Autodesk Fusion 360 part; units mm, degrees
(part 15 of 21)
  spline S63 degree 3 poles (-9.8498, -24.8525) (-9.8587, -24.8489) (-9.8682, -24.8467) (-9.8874, -24.845) (-9.8971, -24.8455) (-9.9193, -24.85) (-9.9314, -24.8551) (-9.9531, -24.8696) (-9.9624, -24.8789) (-9.9696, -24.8897) knots -0.013599 -0.013599 -0.013599 -0.013599 -0.010706 -0.010706 -0.007813 -0.007813 -0.003906 -0.003906 0 0 0 0
  arc A33 (-9.8498, -24.8525) -> (-9.3097, -25.0598) centre (0, 0) ccw
  spline S64 degree 3 poles (-9.2456, -25.1676) (-9.2442, -25.1581) (-9.2442, -25.1484) (-9.2471, -25.1293) (-9.2499, -25.12) (-9.2594, -25.0995) (-9.2672, -25.0888) (-9.2863, -25.0712) (-9.2975, -25.0643) (-9.3097, -25.0598) knots -0.013599 -0.013599 -0.013599 -0.013599 -0.010706 -0.010706 -0.007813 -0.007813 -0.003906 -0.003906 0 0 0 0
  spline S65 degree 3 poles (-9.2557, -27.3039) (-9.2937, -26.9335) (-9.315, -26.5537) (-9.3122, -25.8487) (-9.2928, -25.4995) (-9.2456, -25.1676) knots -0.220678 -0.220678 -0.220678 -0.220678 -0.107909 -0.107909 -0.008028 -0.008028 -0.008028 -0.008028
  arc A34 (-9.2557, -27.3039) -> (-8.5608, -27.5296) centre (0, 0) ccw
  spline S66 degree 3 poles (-7.3133, -25.7954) (-7.4702, -26.0917) (-7.6598, -26.3856) (-8.0719, -26.9576) (-8.3124, -27.2523) (-8.5608, -27.5296) knots -0.210627 -0.210627 -0.210627 -0.210627 -0.111696 -0.111696 0 0 0 0
  spline S67 degree 3 poles (-7.198, -25.7459) (-7.2073, -25.7433) (-7.2169, -25.7421) (-7.2362, -25.7424) (-7.2458, -25.7439) (-7.2674, -25.7508) (-7.2789, -25.757) (-7.2989, -25.7737) (-7.3072, -25.7839) (-7.3133, -25.7954) knots -0.013599 -0.013599 -0.013599 -0.013599 -0.010706 -0.010706 -0.007813 -0.007813 -0.003906 -0.003906 0 0 0 0
  arc A35 (-7.198, -25.7459) -> (-6.6393, -25.8956) centre (0, 0) ccw
  spline S68 degree 3 poles (-6.5642, -25.9962) (-6.5638, -25.9865) (-6.5649, -25.9769) (-6.5697, -25.9582) (-6.5734, -25.9493) (-6.5851, -25.9298) (-6.5939, -25.9201) (-6.6148, -25.9045) (-6.6267, -25.8989) (-6.6393, -25.8956) knots -0.013599 -0.013599 -0.013599 -0.013599 -0.010706 -0.010706 -0.007813 -0.007813 -0.003906 -0.003906 0 0 0 0
  spline S69 degree 3 poles (-6.351, -28.1218) (-6.4275, -27.7574) (-6.4884, -27.3819) (-6.5592, -26.6805) (-6.5765, -26.3312) (-6.5642, -25.9962) knots -0.220678 -0.220678 -0.220678 -0.220678 -0.107909 -0.107909 -0.008028 -0.008028 -0.008028 -0.008028
  arc A36 (-6.351, -28.1218) -> (-5.6363, -28.2737) centre (0, 0) ccw
  spline S70 degree 3 poles (-4.5769, -26.4186) (-4.702, -26.7296) (-4.8598, -27.0417) (-5.2098, -27.6537) (-5.4182, -27.9719) (-5.6363, -28.2737) knots -0.210627 -0.210627 -0.210627 -0.210627 -0.111696 -0.111696 0 0 0 0
  spline S71 degree 3 poles (-4.4674, -26.3573) (-4.4769, -26.3557) (-4.4866, -26.3554) (-4.5058, -26.3578) (-4.5151, -26.3603) (-4.5359, -26.3693) (-4.5467, -26.3768) (-4.5649, -26.3955) (-4.572, -26.4065) (-4.5769, -26.4186) knots -0.013599 -0.013599 -0.013599 -0.013599 -0.010706 -0.010706 -0.007813 -0.007813 -0.003906 -0.003906 0 0 0 0
  arc A37 (-4.4674, -26.3573) -> (-3.8961, -26.4478) centre (0, 0) ccw
  spline S72 degree 3 poles (-3.8109, -26.5399) (-3.8115, -26.5303) (-3.8136, -26.5208) (-3.8203, -26.5027) (-3.825, -26.4942) (-3.8386, -26.4761) (-3.8484, -26.4674) (-3.8708, -26.4541) (-3.8832, -26.4497) (-3.8961, -26.4478) knots -0.013599 -0.013599 -0.013599 -0.013599 -0.010706 -0.010706 -0.007813 -0.007813 -0.003906 -0.003906 0 0 0 0
  spline S73 degree 3 poles (-3.3766, -28.6316) (-3.4908, -28.2772) (-3.5906, -27.9101) (-3.7344, -27.2199) (-3.7881, -26.8744) (-3.8109, -26.5399) knots -0.220678 -0.220678 -0.220678 -0.220678 -0.107909 -0.107909 -0.008028 -0.008028 -0.008028 -0.008028
  arc A38 (-3.3766, -28.6316) -> (-2.65, -28.708) centre (0, 0) ccw
  spline S74 degree 3 poles (-1.7903, -26.7523) (-1.8822, -27.0747) (-2.0065, -27.4015) (-2.2907, -28.0467) (-2.4646, -28.385) (-2.65, -28.708) knots -0.210627 -0.210627 -0.210627 -0.210627 -0.111696 -0.111696 0 0 0 0
  spline S75 degree 3 poles (-1.6879, -26.6799) (-1.6975, -26.6793) (-1.7071, -26.68) (-1.7259, -26.6844) (-1.735, -26.6879) (-1.7547, -26.699) (-1.7647, -26.7076) (-1.7808, -26.728) (-1.7868, -26.7397) (-1.7903, -26.7523) knots -0.013599 -0.013599 -0.013599 -0.013599 -0.010706 -0.010706 -0.007813 -0.007813 -0.003906 -0.003906 0 0 0 0
  arc A39 (-1.6879, -26.6799) -> (-1.1102, -26.7101) centre (0, 0) ccw
  spline S76 degree 3 poles (-1.0158, -26.7929) (-1.0175, -26.7834) (-1.0205, -26.7741) (-1.0291, -26.7569) (-1.0346, -26.7489) (-1.0501, -26.7323) (-1.0607, -26.7246) (-1.0844, -26.7138) (-1.0972, -26.7107) (-1.1102, -26.7101) knots -0.013599 -0.013599 -0.013599 -0.013599 -0.010706 -0.010706 -0.007813 -0.007813 -0.003906 -0.003906 0 0 0 0
  spline S77 degree 3 poles (-0.3653, -28.8277) (-0.5159, -28.4872) (-0.6536, -28.1325) (-0.8687, -27.4612) (-0.9582, -27.1231) (-1.0158, -26.7929) knots -0.220678 -0.220678 -0.220678 -0.220678 -0.107909 -0.107909 -0.008028 -0.008028 -0.008028 -0.008028
  arc A40 (-0.3653, -28.8277) -> (0.3653, -28.8277) centre (0, 0) ccw
  spline S78 degree 3 poles (1.0158, -26.7929) (0.9582, -27.1231) (0.8687, -27.4612) (0.6536, -28.1325) (0.5159, -28.4872) (0.3653, -28.8277) knots -0.210627 -0.210627 -0.210627 -0.210627 -0.111696 -0.111696 0 0 0 0
  spline S79 degree 3 poles (1.1102, -26.7101) (1.1006, -26.7105) (1.091, -26.7123) (1.0728, -26.7186) (1.0642, -26.723) (1.0457, -26.7362) (1.0367, -26.7457) (1.0228, -26.7678) (1.0181, -26.78) (1.0158, -26.7929) knots -0.013599 -0.013599 -0.013599 -0.013599 -0.010706 -0.010706 -0.007813 -0.007813 -0.003906 -0.003906 0 0 0 0
  arc A41 (1.1102, -26.7101) -> (1.6879, -26.6799) centre (0, 0) ccw
  spline S80 degree 3 poles (1.7903, -26.7523) (1.7877, -26.743) (1.7837, -26.7341) (1.7734, -26.7179) (1.7671, -26.7105) (1.75, -26.6957) (1.7386, -26.6891) (1.7139, -26.6808) (1.7008, -26.679) (1.6879, -26.6799) knots -0.013599 -0.013599 -0.013599 -0.013599 -0.010706 -0.010706 -0.007813 -0.007813 -0.003906 -0.003906 0 0 0 0
  spline S81 degree 3 poles (2.65, -28.708) (2.4646, -28.385) (2.2907, -28.0467) (2.0065, -27.4015) (1.8822, -27.0747) (1.7903, -26.7523) knots -0.220678 -0.220678 -0.220678 -0.220678 -0.107909 -0.107909 -0.008028 -0.008028 -0.008028 -0.008028
  arc A42 (2.65, -28.708) -> (3.3766, -28.6316) centre (0, 0) ccw
  spline S82 degree 3 poles (3.8109, -26.5399) (3.7881, -26.8744) (3.7344, -27.2199) (3.5906, -27.9101) (3.4908, -28.2772) (3.3766, -28.6316) knots -0.210627 -0.210627 -0.210627 -0.210627 -0.111696 -0.111696 0 0 0 0
  spline S83 degree 3 poles (3.8961, -26.4478) (3.8865, -26.4492) (3.8773, -26.452) (3.8598, -26.4601) (3.8517, -26.4654) (3.8347, -26.4804) (3.8267, -26.4908) (3.8152, -26.5142) (3.8118, -26.5269) (3.8109, -26.5399) knots -0.013599 -0.013599 -0.013599 -0.013599 -0.010706 -0.010706 -0.007813 -0.007813 -0.003906 -0.003906 0 0 0 0
  arc A43 (3.8961, -26.4478) -> (4.4674, -26.3573) centre (0, 0) ccw
  spline S84 degree 3 poles (4.5769, -26.4186) (4.5733, -26.4096) (4.5684, -26.4012) (4.5564, -26.3861) (4.5494, -26.3795) (4.5308, -26.3665) (4.5188, -26.3612) (4.4934, -26.3555) (4.4803, -26.3551) (4.4674, -26.3573) knots -0.013599 -0.013599 -0.013599 -0.013599 -0.010706 -0.010706 -0.007813 -0.007813 -0.003906 -0.003906 0 0 0 0
  spline S85 degree 3 poles (5.6363, -28.2737) (5.4182, -27.9719) (5.2098, -27.6537) (4.8598, -27.0417) (4.702, -26.7296) (4.5769, -26.4186) knots -0.220678 -0.220678 -0.220678 -0.220678 -0.107909 -0.107909 -0.008028 -0.008028 -0.008028 -0.008028
  arc A44 (5.6363, -28.2737) -> (6.351, -28.1218) centre (0, 0) ccw
  spline S86 degree 3 poles (6.5642, -25.9962) (6.5765, -26.3312) (6.5592, -26.6805) (6.4884, -27.3819) (6.4275, -27.7574) (6.351, -28.1218) knots -0.210627 -0.210627 -0.210627 -0.210627 -0.111696 -0.111696 0 0 0 0
  spline S87 degree 3 poles (6.6393, -25.8956) (6.6299, -25.898) (6.621, -25.9018) (6.6045, -25.9117) (6.5969, -25.9178) (6.5816, -25.9345) (6.5748, -25.9457) (6.5658, -25.9702) (6.5637, -25.9831) (6.5642, -25.9962) knots -0.013599 -0.013599 -0.013599 -0.013599 -0.010706 -0.010706 -0.007813 -0.007813 -0.003906 -0.003906 0 0 0 0
  arc A45 (6.6393, -25.8956) -> (7.198, -25.7459) centre (0, 0) ccw
  spline S88 degree 3 poles (7.3133, -25.7954) (7.3088, -25.7869) (7.3031, -25.7791) (7.2896, -25.7653) (7.2819, -25.7594) (7.2621, -25.7485) (7.2495, -25.7444) (7.2237, -25.7414) (7.2106, -25.7424) (7.198, -25.7459) knots -0.013599 -0.013599 -0.013599 -0.013599 -0.010706 -0.010706 -0.007813 -0.007813 -0.003906 -0.003906 0 0 0 0
  spline S89 degree 3 poles (8.5608, -27.5296) (8.3124, -27.2523) (8.0719, -26.9576) (7.6598, -26.3856) (7.4702, -26.0917) (7.3133, -25.7954) knots -0.220678 -0.220678 -0.220678 -0.220678 -0.107909 -0.107909 -0.008028 -0.008028 -0.008028 -0.008028
  arc A46 (8.5608, -27.5296) -> (9.2557, -27.3039) centre (0, 0) ccw
  spline S90 degree 3 poles (9.2456, -25.1676) (9.2928, -25.4995) (9.3122, -25.8487) (9.315, -26.5537) (9.2937, -26.9335) (9.2557, -27.3039) knots -0.210627 -0.210627 -0.210627 -0.210627 -0.111696 -0.111696 0 0 0 0
  spline S91 degree 3 poles (9.3097, -25.0598) (9.3007, -25.0631) (9.2922, -25.0678) (9.2768, -25.0794) (9.27, -25.0863) (9.2565, -25.1045) (9.2508, -25.1163) (9.2444, -25.1416) (9.2437, -25.1547) (9.2456, -25.1676) knots -0.013599 -0.013599 -0.013599 -0.013599 -0.010706 -0.010706 -0.007813 -0.007813 -0.003906 -0.003906 0 0 0 0
  arc A47 (9.3097, -25.0598) -> (9.8498, -24.8525) centre (0, 0) ccw
  spline S92 degree 3 poles (9.9696, -24.8897) (9.9642, -24.8817) (9.9577, -24.8745) (9.9429, -24.8622) (9.9346, -24.8572) (9.9137, -24.8483) (9.9008, -24.8456) (9.8748, -24.8453) (9.8619, -24.8477) (9.8498, -24.8525) knots -0.013599 -0.013599 -0.013599 -0.013599 -0.010706 -0.010706 -0.007813 -0.007813 -0.003906 -0.003906 0 0 0 0
  spline S93 degree 3 poles (11.3915, -26.484) (11.1155, -26.2342) (10.8455, -25.9662) (10.3759, -25.4404) (10.1566, -25.1679) (9.9696, -24.8897) knots -0.220678 -0.220678 -0.220678 -0.220678 -0.107909 -0.107909 -0.008028 -0.008028 -0.008028 -0.008028
  arc A48 (11.3915, -26.484) -> (12.059, -26.1868) centre (0, 0) ccw
  spline S94 degree 3 poles (11.8257, -24.0633) (11.9073, -24.3884) (11.9631, -24.7337) (12.0396, -25.4345) (12.0581, -25.8145) (12.059, -26.1868) knots -0.210627 -0.210627 -0.210627 -0.210627 -0.111696 -0.111696 0 0 0 0
  spline S95 degree 3 poles (11.8782, -23.9494) (11.8696, -23.9537) (11.8616, -23.9592) (11.8475, -23.9723) (11.8414, -23.9799) (11.8299, -23.9994) (11.8255, -24.0118) (11.8218, -24.0376) (11.8225, -24.0507) (11.8257, -24.0633) knots -0.013599 -0.013599 -0.013599 -0.013599 -0.010706 -0.010706 -0.007813 -0.007813 -0.003906 -0.003906 0 0 0 0
  arc A49 (11.8782, -23.9494) -> (12.3936, -23.6868) centre (0, 0) ccw
  spline S96 degree 3 poles (12.5167, -23.7112) (12.5105, -23.7038) (12.5033, -23.6974) (12.4872, -23.6867) (12.4784, -23.6826) (12.4568, -23.6759) (12.4437, -23.6746) (12.4178, -23.677) (12.4051, -23.6807) (12.3936, -23.6868) knots -0.013599 -0.013599 -0.013599 -0.013599 -0.010706 -0.010706 -0.007813 -0.007813 -0.003906 -0.003906 0 0 0 0
  spline S97 degree 3 poles (14.0975, -25.1482) (13.7968, -24.9286) (13.5003, -24.6903) (12.9783, -24.2164) (12.7317, -23.9684) (12.5167, -23.7112) knots -0.220678 -0.220678 -0.220678 -0.220678 -0.107909 -0.107909 -0.008028 -0.008028 -0.008028 -0.008028
  arc A50 (14.0975, -25.1482) -> (14.7302, -24.7828) centre (0, 0) ccw
  spline S98 degree 3 poles (14.2762, -22.6954) (14.3914, -23.0102) (14.4829, -23.3477) (14.6323, -24.0367) (14.6904, -24.4127) (14.7302, -24.7828) knots -0.210627 -0.210627 -0.210627 -0.210627 -0.111696 -0.111696 0 0 0 0
  spline S99 degree 3 poles (14.3165, -22.5766) (14.3084, -22.5817) (14.301, -22.588) (14.2884, -22.6026) (14.2831, -22.6107) (14.2737, -22.6313) (14.2707, -22.6441) (14.2697, -22.6702) (14.2717, -22.6831) (14.2762, -22.6954) knots -0.013599 -0.013599 -0.013599 -0.013599 -0.010706 -0.010706 -0.007813 -0.007813 -0.003906 -0.003906 0 0 0 0
  arc A51 (14.3165, -22.5766) -> (14.8017, -22.2615) centre (0, 0) ccw
  spline S100 degree 3 poles (14.9266, -22.273) (14.9197, -22.2663) (14.9118, -22.2606) (14.8947, -22.2517) (14.8856, -22.2485) (14.8633, -22.2441) (14.8502, -22.2442) (14.8246, -22.2493) (14.8125, -22.2543) (14.8017, -22.2615) knots -0.013599 -0.013599 -0.013599 -0.013599 -0.010706 -0.010706 -0.007813 -0.007813 -0.003906 -0.003906 0 0 0 0
  spline S101 degree 3 poles (16.6489, -23.5368) (16.327, -23.3499) (16.0071, -23.1439) (15.4385, -22.7272) (15.1674, -22.5063) (14.9266, -22.273) knots -0.220678 -0.220678 -0.220678 -0.220678 -0.107909 -0.107909 -0.008028 -0.008028 -0.008028 -0.008028
  arc A52 (16.6489, -23.5368) -> (17.24, -23.1074) centre (0, 0) ccw
  spline S102 degree 3 poles (16.5703, -21.0788) (16.7177, -21.3798) (16.8441, -21.7059) (17.0646, -22.3755) (17.1617, -22.7434) (17.24, -23.1074) knots -0.210627 -0.210627 -0.210627 -0.210627 -0.111696 -0.111696 0 0 0 0
  spline S103 degree 3 poles (16.598, -20.9564) (16.5904, -20.9624) (16.5838, -20.9694) (16.5727, -20.9852) (16.5683, -20.9939) (16.5611, -21.0154) (16.5594, -21.0284) (16.5612, -21.0544) (16.5645, -21.0671) (16.5703, -21.0788) knots -0.013599 -0.013599 -0.013599 -0.013599 -0.010706 -0.010706 -0.007813 -0.007813 -0.003906 -0.003906 0 0 0 0
  arc A53 (16.598, -20.9564) -> (17.0475, -20.5924) centre (0, 0) ccw
  spline S104 degree 3 poles (17.173, -20.5907) (17.1654, -20.5848) (17.157, -20.5799) (17.1391, -20.5728) (17.1296, -20.5706) (17.1071, -20.5686) (17.094, -20.5701) (17.0691, -20.5778) (17.0576, -20.5841) (17.0475, -20.5924) knots -0.013599 -0.013599 -0.013599 -0.013599 -0.010706 -0.010706 -0.007813 -0.007813 -0.003906 -0.003906 0 0 0 0
  spline S105 degree 3 poles (19.018, -21.6676) (18.6782, -21.5153) (18.3387, -21.3439) (17.7295, -20.9889) (17.4368, -20.7975) (17.173, -20.5907) knots -0.220678 -0.220678 -0.220678 -0.220678 -0.107909 -0.107909 -0.008028 -0.008028 -0.008028 -0.008028
  arc A54 (19.018, -21.6676) -> (19.561, -21.1787) centre (0, 0) ccw
  spline S106 degree 3 poles (18.6828, -19.2312) (18.861, -19.5152) (19.0207, -19.8263) (19.31, -20.4692) (19.445, -20.8249) (19.561, -21.1787) knots -0.210627 -0.210627 -0.210627 -0.210627 -0.111696 -0.111696 0 0 0 0
  spline S107 degree 3 poles (18.6976, -19.1066) (18.6907, -19.1134) (18.6848, -19.1211) (18.6755, -19.1379) (18.672, -19.147) (18.6671, -19.1691) (18.6668, -19.1823) (18.6712, -19.2079) (18.6759, -19.2202) (18.6828, -19.2312) knots -0.013599 -0.013599 -0.013599 -0.013599 -0.010706 -0.010706 -0.007813 -0.007813 -0.003906 -0.003906 0 0 0 0
  arc A55 (18.6976, -19.1066) -> (19.1066, -18.6976) centre (0, 0) ccw
  spline S108 degree 3 poles (19.2312, -18.6828) (19.2231, -18.6777) (19.2142, -18.6738) (19.1956, -18.6686) (19.186, -18.6674) (19.1633, -18.6678) (19.1505, -18.6706) (19.1266, -18.6809) (19.1157, -18.6883) (19.1066, -18.6976) knots -0.013599 -0.013599 -0.013599 -0.013599 -0.010706 -0.010706 -0.007813 -0.007813 -0.003906 -0.003906 0 0 0 0
  spline S109 degree 3 poles (21.1787, -19.561) (20.8249, -19.445) (20.4692, -19.31) (19.8263, -19.0207) (19.5152, -18.861) (19.2312, -18.6828) knots -0.220678 -0.220678 -0.220678 -0.220678 -0.107909 -0.107909 -0.008028 -0.008028 -0.008028 -0.008028
  arc A56 (21.1787, -19.561) -> (21.6676, -19.018) centre (0, 0) ccw
  spline S110 degree 3 poles (20.5907, -17.173) (20.7975, -17.4368) (20.9889, -17.7295) (21.3439, -18.3387) (21.5153, -18.6782) (21.6676, -19.018) knots -0.210627 -0.210627 -0.210627 -0.210627 -0.111696 -0.111696 0 0 0 0
  spline S111 degree 3 poles (20.5924, -17.0475) (20.5862, -17.055) (20.5812, -17.0632) (20.5736, -17.081) (20.5711, -17.0904) (20.5686, -17.1129) (20.5696, -17.126) (20.5767, -17.151) (20.5827, -17.1628) (20.5907, -17.173) knots -0.013599 -0.013599 -0.013599 -0.013599 -0.010706 -0.010706 -0.007813 -0.007813 -0.003906 -0.003906 0 0 0 0
  arc A57 (20.5924, -17.0475) -> (20.9564, -16.598) centre (0, 0) ccw
  spline S112 degree 3 poles (21.0788, -16.5703) (21.0701, -16.566) (21.0609, -16.5631) (21.0419, -16.5599) (21.0322, -16.5597) (21.0097, -16.5624) (20.9972, -16.5665) (20.9745, -16.5793) (20.9645, -16.5878) (20.9564, -16.598) knots -0.013599 -0.013599 -0.013599 -0.013599 -0.010706 -0.010706 -0.007813 -0.007813 -0.003906 -0.003906 0 0 0 0
  spline S113 degree 3 poles (23.1074, -17.24) (22.7434, -17.1617) (22.3755, -17.0646) (21.7059, -16.8441) (21.3798, -16.7177) (21.0788, -16.5703) knots -0.220678 -0.220678 -0.220678 -0.220678 -0.107909 -0.107909 -0.008028 -0.008028 -0.008028 -0.008028
  arc A58 (23.1074, -17.24) -> (23.5368, -16.6489) centre (0, 0) ccw
  spline S114 degree 3 poles (22.273, -14.9266) (22.5063, -15.1674) (22.7272, -15.4385) (23.1439, -16.0071) (23.3499, -16.327) (23.5368, -16.6489) knots -0.210627 -0.210627 -0.210627 -0.210627 -0.111696 -0.111696 0 0 0 0
  spline S115 degree 3 poles (22.2615, -14.8017) (22.2562, -14.8097) (22.252, -14.8184) (22.2464, -14.8369) (22.2449, -14.8465) (22.2447, -14.8691) (22.2471, -14.882) (22.2568, -14.9062) (22.2639, -14.9173) (22.273, -14.9266) knots -0.013599 -0.013599 -0.013599 -0.013599 -0.010706 -0.010706 -0.007813 -0.007813 -0.003906 -0.003906 0 0 0 0
  arc A59 (22.2615, -14.8017) -> (22.5766, -14.3165) centre (0, 0) ccw
  spline S116 degree 3 poles (22.6954, -14.2762) (22.6863, -14.2729) (22.6768, -14.2709) (22.6576, -14.2697) (22.6479, -14.2705) (22.6258, -14.2756) (22.6138, -14.2809) (22.5926, -14.296) (22.5835, -14.3055) (22.5766, -14.3165) knots -0.013599 -0.013599 -0.013599 -0.013599 -0.010706 -0.010706 -0.007813 -0.007813 -0.003906 -0.003906 0 0 0 0
  spline S117 degree 3 poles (24.7828, -14.7302) (24.4127, -14.6904) (24.0367, -14.6323) (23.3477, -14.4829) (23.0102, -14.3914) (22.6954, -14.2762) knots -0.220678 -0.220678 -0.220678 -0.220678 -0.107909 -0.107909 -0.008028 -0.008028 -0.008028 -0.008028
  arc A60 (24.7828, -14.7302) -> (25.1482, -14.0975) centre (0, 0) ccw
  spline S118 degree 3 poles (23.7112, -12.5167) (23.9684, -12.7317) (24.2164, -12.9783) (24.6903, -13.5003) (24.9286, -13.7968) (25.1482, -14.0975) knots -0.210627 -0.210627 -0.210627 -0.210627 -0.111696 -0.111696 0 0 0 0
  spline S119 degree 3 poles (23.6868, -12.3936) (23.6823, -12.4022) (23.6791, -12.4113) (23.6754, -12.4302) (23.6749, -12.4399) (23.6771, -12.4625) (23.6808, -12.4751) (23.693, -12.4981) (23.7012, -12.5083) (23.7112, -12.5167) knots -0.013599 -0.013599 -0.013599 -0.013599 -0.010706 -0.010706 -0.007813 -0.007813 -0.003906 -0.003906 0 0 0 0
  arc A61 (23.6868, -12.3936) -> (23.9494, -11.8782) centre (0, 0) ccw
  spline S120 degree 3 poles (24.0633, -11.8257) (24.054, -11.8233) (24.0443, -11.8223) (24.025, -11.8231) (24.0155, -11.8249) (23.9941, -11.8323) (23.9827, -11.8389) (23.9632, -11.8561) (23.9552, -11.8665) (23.9494, -11.8782) knots -0.013599 -0.013599 -0.013599 -0.013599 -0.010706 -0.010706 -0.007813 -0.007813 -0.003906 -0.003906 0 0 0 0
  spline S121 degree 3 poles (26.1868, -12.059) (25.8145, -12.0581) (25.4345, -12.0396) (24.7337, -11.9631) (24.3884, -11.9073) (24.0633, -11.8257) knots -0.220678 -0.220678 -0.220678 -0.220678 -0.107909 -0.107909 -0.008028 -0.008028 -0.008028 -0.008028
  arc A62 (26.1868, -12.059) -> (26.484, -11.3915) centre (0, 0) ccw
  spline S122 degree 3 poles (24.8897, -9.9696) (25.1679, -10.1566) (25.4404, -10.3759) (25.9662, -10.8455) (26.2342, -11.1155) (26.484, -11.3915) knots -0.210627 -0.210627 -0.210627 -0.210627 -0.111696 -0.111696 0 0 0 0
  spline S123 degree 3 poles (24.8525, -9.8498) (24.8489, -9.8587) (24.8467, -9.8682) (24.845, -9.8874) (24.8455, -9.8971) (24.85, -9.9193) (24.8551, -9.9314) (24.8696, -9.9531) (24.8789, -9.9624) (24.8897, -9.9696) knots -0.013599 -0.013599 -0.013599 -0.013599 -0.010706 -0.010706 -0.007813 -0.007813 -0.003906 -0.003906 0 0 0 0
  arc A63 (24.8525, -9.8498) -> (25.0598, -9.3097) centre (0, 0) ccw
  spline S124 degree 3 poles (25.1676, -9.2456) (25.1581, -9.2442) (25.1484, -9.2442) (25.1293, -9.2471) (25.12, -9.2499) (25.0995, -9.2594) (25.0888, -9.2672) (25.0712, -9.2863) (25.0643, -9.2975) (25.0598, -9.3097) knots -0.013599 -0.013599 -0.013599 -0.013599 -0.010706 -0.010706 -0.007813 -0.007813 -0.003906 -0.003906 0 0 0 0
  spline S125 degree 3 poles (27.3039, -9.2557) (26.9335, -9.2937) (26.5537, -9.315) (25.8487, -9.3122) (25.4995, -9.2928) (25.1676, -9.2456) knots -0.220678 -0.220678 -0.220678 -0.220678 -0.107909 -0.107909 -0.008028 -0.008028 -0.008028 -0.008028
  arc A64 (27.3039, -9.2557) -> (27.5296, -8.5608) centre (0, 0) ccw
  spline S126 degree 3 poles (25.7954, -7.3133) (26.0917, -7.4702) (26.3856, -7.6598) (26.9576, -8.0719) (27.2523, -8.3124) (27.5296, -8.5608) knots -0.210627 -0.210627 -0.210627 -0.210627 -0.111696 -0.111696 0 0 0 0
  spline S127 degree 3 poles (25.7459, -7.198) (25.7433, -7.2073) (25.7421, -7.2169) (25.7424, -7.2362) (25.7439, -7.2458) (25.7508, -7.2674) (25.757, -7.2789) (25.7737, -7.2989) (25.7839, -7.3072) (25.7954, -7.3133) knots -0.013599 -0.013599 -0.013599 -0.013599 -0.010706 -0.010706 -0.007813 -0.007813 -0.003906 -0.003906 0 0 0 0
  arc A65 (25.7459, -7.198) -> (25.8956, -6.6393) centre (0, 0) ccw
  spline S128 degree 3 poles (25.9962, -6.5642) (25.9865, -6.5638) (25.9769, -6.5649) (25.9582, -6.5697) (25.9493, -6.5734) (25.9298, -6.5851) (25.9201, -6.5939) (25.9045, -6.6148) (25.8989, -6.6267) (25.8956, -6.6393) knots -0.013599 -0.013599 -0.013599 -0.013599 -0.010706 -0.010706 -0.007813 -0.007813 -0.003906 -0.003906 0 0 0 0
  spline S129 degree 3 poles (28.1218, -6.351) (27.7574, -6.4275) (27.3819, -6.4884) (26.6805, -6.5592) (26.3312, -6.5765) (25.9962, -6.5642) knots -0.220678 -0.220678 -0.220678 -0.220678 -0.107909 -0.107909 -0.008028 -0.008028 -0.008028 -0.008028
  arc A66 (28.1218, -6.351) -> (28.2737, -5.6363) centre (0, 0) ccw
  spline S130 degree 3 poles (26.4186, -4.5769) (26.7296, -4.702) (27.0417, -4.8598) (27.6537, -5.2098) (27.9719, -5.4182) (28.2737, -5.6363) knots -0.210627 -0.210627 -0.210627 -0.210627 -0.111696 -0.111696 0 0 0 0
  spline S131 degree 3 poles (26.3573, -4.4674) (26.3557, -4.4769) (26.3554, -4.4866) (26.3578, -4.5058) (26.3603, -4.5151) (26.3693, -4.5359) (26.3768, -4.5467) (26.3955, -4.5649) (26.4065, -4.572) (26.4186, -4.5769) knots -0.013599 -0.013599 -0.013599 -0.013599 -0.010706 -0.010706 -0.007813 -0.007813 -0.003906 -0.003906 0 0 0 0
  arc A67 (26.3573, -4.4674) -> (26.4478, -3.8961) centre (0, 0) ccw
  spline S132 degree 3 poles (26.5399, -3.8109) (26.5303, -3.8115) (26.5208, -3.8136) (26.5027, -3.8203) (26.4942, -3.825) (26.4761, -3.8386) (26.4674, -3.8484) (26.4541, -3.8708) (26.4497, -3.8832) (26.4478, -3.8961) knots -0.013599 -0.013599 -0.013599 -0.013599 -0.010706 -0.010706 -0.007813 -0.007813 -0.003906 -0.003906 0 0 0 0
  spline S133 degree 3 poles (28.6316, -3.3766) (28.2772, -3.4908) (27.9101, -3.5906) (27.2199, -3.7344) (26.8744, -3.7881) (26.5399, -3.8109) knots -0.220678 -0.220678 -0.220678 -0.220678 -0.107909 -0.107909 -0.008028 -0.008028 -0.008028 -0.008028
  arc A68 (28.6316, -3.3766) -> (28.708, -2.65) centre (0, 0) ccw
  spline S134 degree 3 poles (26.7523, -1.7903) (27.0747, -1.8822) (27.4015, -2.0065) (28.0467, -2.2907) (28.385, -2.4646) (28.708, -2.65) knots -0.210627 -0.210627 -0.210627 -0.210627 -0.111696 -0.111696 0 0 0 0
  spline S135 degree 3 poles (26.6799, -1.6879) (26.6793, -1.6975) (26.68, -1.7071) (26.6844, -1.7259) (26.6879, -1.735) (26.699, -1.7547) (26.7076, -1.7647) (26.728, -1.7808) (26.7397, -1.7868) (26.7523, -1.7903) knots -0.013599 -0.013599 -0.013599 -0.013599 -0.010706 -0.010706 -0.007813 -0.007813 -0.003906 -0.003906 0 0 0 0
  arc A69 (26.6799, -1.6879) -> (26.7101, -1.1102) centre (0, 0) ccw
  spline S136 degree 3 poles (26.7929, -1.0158) (26.7834, -1.0175) (26.7741, -1.0205) (26.7569, -1.0291) (26.7489, -1.0346) (26.7323, -1.0501) (26.7246, -1.0607) (26.7138, -1.0844) (26.7107, -1.0972) (26.7101, -1.1102) knots -0.013599 -0.013599 -0.013599 -0.013599 -0.010706 -0.010706 -0.007813 -0.007813 -0.003906 -0.003906 0 0 0 0
  spline S137 degree 3 poles (28.8277, -0.3653) (28.4872, -0.5159) (28.1325, -0.6536) (27.4612, -0.8687) (27.1231, -0.9582) (26.7929, -1.0158) knots -0.220678 -0.220678 -0.220678 -0.220678 -0.107909 -0.107909 -0.008028 -0.008028 -0.008028 -0.008028
  arc A70 (28.8277, -0.3653) -> (28.8277, 0.3653) centre (0, 0) ccw
  spline S138 degree 3 poles (26.7929, 1.0158) (27.1231, 0.9582) (27.4612, 0.8687) (28.1325, 0.6536) (28.4872, 0.5159) (28.8277, 0.3653) knots -0.210627 -0.210627 -0.210627 -0.210627 -0.111696 -0.111696 0 0 0 0
  spline S139 degree 3 poles (26.7101, 1.1102) (26.7105, 1.1006) (26.7123, 1.091) (26.7186, 1.0728) (26.723, 1.0642) (26.7362, 1.0457) (26.7457, 1.0367) (26.7678, 1.0228) (26.78, 1.0181) (26.7929, 1.0158) knots -0.013599 -0.013599 -0.013599 -0.013599 -0.010706 -0.010706 -0.007813 -0.007813 -0.003906 -0.003906 0 0 0 0
  arc A71 (26.7101, 1.1102) -> (26.6799, 1.6879) centre (0, 0) ccw
  spline S140 degree 3 poles (26.7523, 1.7903) (26.743, 1.7877) (26.7341, 1.7837) (26.7179, 1.7734) (26.7105, 1.7671) (26.6957, 1.75) (26.6891, 1.7386) (26.6808, 1.7139) (26.679, 1.7008) (26.6799, 1.6879) knots -0.013599 -0.013599 -0.013599 -0.013599 -0.010706 -0.010706 -0.007813 -0.007813 -0.003906 -0.003906 0 0 0 0
  spline S141 degree 3 poles (28.708, 2.65) (28.385, 2.4646) (28.0467, 2.2907) (27.4015, 2.0065) (27.0747, 1.8822) (26.7523, 1.7903) knots -0.220678 -0.220678 -0.220678 -0.220678 -0.107909 -0.107909 -0.008028 -0.008028 -0.008028 -0.008028
  arc A72 (28.708, 2.65) -> (28.6316, 3.3766) centre (0, 0) ccw
  spline S142 degree 3 poles (26.5399, 3.8109) (26.8744, 3.7881) (27.2199, 3.7344) (27.9101, 3.5906) (28.2772, 3.4908) (28.6316, 3.3766) knots -0.210627 -0.210627 -0.210627 -0.210627 -0.111696 -0.111696 0 0 0 0
  spline S143 degree 3 poles (26.4478, 3.8961) (26.4492, 3.8865) (26.452, 3.8773) (26.4601, 3.8598) (26.4654, 3.8517) (26.4804, 3.8347) (26.4908, 3.8267) (26.5142, 3.8152) (26.5269, 3.8118) (26.5399, 3.8109) knots -0.013599 -0.013599 -0.013599 -0.013599 -0.010706 -0.010706 -0.007813 -0.007813 -0.003906 -0.003906 0 0 0 0
  arc A73 (26.4478, 3.8961) -> (26.3573, 4.4674) centre (0, 0) ccw
  spline S144 degree 3 poles (26.4186, 4.5769) (26.4096, 4.5733) (26.4012, 4.5684) (26.3861, 4.5564) (26.3795, 4.5494) (26.3665, 4.5308) (26.3612, 4.5188) (26.3555, 4.4934) (26.3551, 4.4803) (26.3573, 4.4674) knots -0.013599 -0.013599 -0.013599 -0.013599 -0.010706 -0.010706 -0.007813 -0.007813 -0.003906 -0.003906 0 0 0 0
  spline S145 degree 3 poles (28.2737, 5.6363) (27.9719, 5.4182) (27.6537, 5.2098) (27.0417, 4.8598) (26.7296, 4.702) (26.4186, 4.5769) knots -0.220678 -0.220678 -0.220678 -0.220678 -0.107909 -0.107909 -0.008028 -0.008028 -0.008028 -0.008028
  arc A74 (28.2737, 5.6363) -> (28.1218, 6.351) centre (0, 0) ccw
  spline S146 degree 3 poles (25.9962, 6.5642) (26.3312, 6.5765) (26.6805, 6.5592) (27.3819, 6.4884) (27.7574, 6.4275) (28.1218, 6.351) knots -0.210627 -0.210627 -0.210627 -0.210627 -0.111696 -0.111696 0 0 0 0
  spline S147 degree 3 poles (25.8956, 6.6393) (25.898, 6.6299) (25.9018, 6.621) (25.9117, 6.6045) (25.9178, 6.5969) (25.9345, 6.5816) (25.9457, 6.5748) (25.9702, 6.5658) (25.9831, 6.5637) (25.9962, 6.5642) knots -0.013599 -0.013599 -0.013599 -0.013599 -0.010706 -0.010706 -0.007813 -0.007813 -0.003906 -0.003906 0 0 0 0
  arc A75 (25.8956, 6.6393) -> (25.7459, 7.198) centre (0, 0) ccw
  spline S148 degree 3 poles (25.7954, 7.3133) (25.7869, 7.3088) (25.7791, 7.3031) (25.7653, 7.2896) (25.7594, 7.2819) (25.7485, 7.2621) (25.7444, 7.2495) (25.7414, 7.2237) (25.7424, 7.2106) (25.7459, 7.198) knots -0.013599 -0.013599 -0.013599 -0.013599 -0.010706 -0.010706 -0.007813 -0.007813 -0.003906 -0.003906 0 0 0 0
  spline S149 degree 3 poles (27.5296, 8.5608) (27.2523, 8.3124) (26.9576, 8.0719) (26.3856, 7.6598) (26.0917, 7.4702) (25.7954, 7.3133) knots -0.220678 -0.220678 -0.220678 -0.220678 -0.107909 -0.107909 -0.008028 -0.008028 -0.008028 -0.008028
  arc A76 (27.5296, 8.5608) -> (27.3039, 9.2557) centre (0, 0) ccw
  spline S150 degree 3 poles (25.1676, 9.2456) (25.4995, 9.2928) (25.8487, 9.3122) (26.5537, 9.315) (26.9335, 9.2937) (27.3039, 9.2557) knots -0.210627 -0.210627 -0.210627 -0.210627 -0.111696 -0.111696 0 0 0 0
  spline S151 degree 3 poles (25.0598, 9.3097) (25.0631, 9.3007) (25.0678, 9.2922) (25.0794, 9.2768) (25.0863, 9.27) (25.1045, 9.2565) (25.1163, 9.2508) (25.1416, 9.2444) (25.1547, 9.2437) (25.1676, 9.2456) knots -0.013599 -0.013599 -0.013599 -0.013599 -0.010706 -0.010706 -0.007813 -0.007813 -0.003906 -0.003906 0 0 0 0
  arc A77 (25.0598, 9.3097) -> (24.8525, 9.8498) centre (0, 0) ccw
  spline S152 degree 3 poles (24.8897, 9.9696) (24.8817, 9.9642) (24.8745, 9.9577) (24.8622, 9.9429) (24.8572, 9.9346) (24.8483, 9.9137) (24.8456, 9.9008) (24.8453, 9.8748) (24.8477, 9.8619) (24.8525, 9.8498) knots -0.013599 -0.013599 -0.013599 -0.013599 -0.010706 -0.010706 -0.007813 -0.007813 -0.003906 -0.003906 0 0 0 0
  spline S153 degree 3 poles (26.484, 11.3915) (26.2342, 11.1155) (25.9662, 10.8455) (25.4404, 10.3759) (25.1679, 10.1566) (24.8897, 9.9696) knots -0.220678 -0.220678 -0.220678 -0.220678 -0.107909 -0.107909 -0.008028 -0.008028 -0.008028 -0.008028
  arc A78 (26.484, 11.3915) -> (26.1868, 12.059) centre (0, 0) ccw
  spline S154 degree 3 poles (24.0633, 11.8257) (24.3884, 11.9073) (24.7337, 11.9631) (25.4345, 12.0396) (25.8145, 12.0581) (26.1868, 12.059) knots -0.210627 -0.210627 -0.210627 -0.210627 -0.111696 -0.111696 0 0 0 0
  spline S155 degree 3 poles (23.9494, 11.8782) (23.9537, 11.8696) (23.9592, 11.8616) (23.9723, 11.8475) (23.9799, 11.8414) (23.9994, 11.8299) (24.0118, 11.8255) (24.0376, 11.8218) (24.0507, 11.8225) (24.0633, 11.8257) knots -0.013599 -0.013599 -0.013599 -0.013599 -0.010706 -0.010706 -0.007813 -0.007813 -0.003906 -0.003906 0 0 0 0
  arc A79 (23.9494, 11.8782) -> (23.6868, 12.3936) centre (0, 0) ccw
  spline S156 degree 3 poles (23.7112, 12.5167) (23.7038, 12.5105) (23.6974, 12.5033) (23.6867, 12.4872) (23.6826, 12.4784) (23.6759, 12.4568) (23.6746, 12.4437) (23.677, 12.4178) (23.6807, 12.4051) (23.6868, 12.3936) knots -0.013599 -0.013599 -0.013599 -0.013599 -0.010706 -0.010706 -0.007813 -0.007813 -0.003906 -0.003906 0 0 0 0
  spline S157 degree 3 poles (25.1482, 14.0975) (24.9286, 13.7968) (24.6903, 13.5003) (24.2164, 12.9783) (23.9684, 12.7317) (23.7112, 12.5167) knots -0.220678 -0.220678 -0.220678 -0.220678 -0.107909 -0.107909 -0.008028 -0.008028 -0.008028 -0.008028
  arc A80 (25.1482, 14.0975) -> (24.7828, 14.7302) centre (0, 0) ccw
  spline S158 degree 3 poles (22.6954, 14.2762) (23.0102, 14.3914) (23.3477, 14.4829) (24.0367, 14.6323) (24.4127, 14.6904) (24.7828, 14.7302) knots -0.210627 -0.210627 -0.210627 -0.210627 -0.111696 -0.111696 0 0 0 0
  spline S159 degree 3 poles (22.5766, 14.3165) (22.5817, 14.3084) (22.588, 14.301) (22.6026, 14.2884) (22.6107, 14.2831) (22.6313, 14.2737) (22.6441, 14.2707) (22.6702, 14.2697) (22.6831, 14.2717) (22.6954, 14.2762) knots -0.013599 -0.013599 -0.013599 -0.013599 -0.010706 -0.010706 -0.007813 -0.007813 -0.003906 -0.003906 0 0 0 0
  arc A81 (22.5766, 14.3165) -> (22.2615, 14.8017) centre (0, 0) ccw
  spline S160 degree 3 poles (22.273, 14.9266) (22.2663, 14.9197) (22.2606, 14.9118) (22.2517, 14.8947) (22.2485, 14.8856) (22.2441, 14.8633) (22.2442, 14.8502) (22.2493, 14.8246) (22.2543, 14.8125) (22.2615, 14.8017) knots -0.013599 -0.013599 -0.013599 -0.013599 -0.010706 -0.010706 -0.007813 -0.007813 -0.003906 -0.003906 0 0 0 0
  spline S161 degree 3 poles (23.5368, 16.6489) (23.3499, 16.327) (23.1439, 16.0071) (22.7272, 15.4385) (22.5063, 15.1674) (22.273, 14.9266) knots -0.220678 -0.220678 -0.220678 -0.220678 -0.107909 -0.107909 -0.008028 -0.008028 -0.008028 -0.008028
  arc A82 (23.5368, 16.6489) -> (23.1074, 17.24) centre (0, 0) ccw
  spline S162 degree 3 poles (21.0788, 16.5703) (21.3798, 16.7177) (21.7059, 16.8441) (22.3755, 17.0646) (22.7434, 17.1617) (23.1074, 17.24) knots -0.210627 -0.210627 -0.210627 -0.210627 -0.111696 -0.111696 0 0 0 0
  spline S163 degree 3 poles (20.9564, 16.598) (20.9624, 16.5904) (20.9694, 16.5838) (20.9852, 16.5727) (20.9939, 16.5683) (21.0154, 16.5611) (21.0284, 16.5594) (21.0544, 16.5612) (21.0671, 16.5645) (21.0788, 16.5703) knots -0.013599 -0.013599 -0.013599 -0.013599 -0.010706 -0.010706 -0.007813 -0.007813 -0.003906 -0.003906 0 0 0 0
  arc A83 (20.9564, 16.598) -> (20.5924, 17.0475) centre (0, 0) ccw
  spline S164 degree 3 poles (20.5907, 17.173) (20.5848, 17.1654) (20.5799, 17.157) (20.5728, 17.1391) (20.5706, 17.1296) (20.5686, 17.1071) (20.5701, 17.094) (20.5778, 17.0691) (20.5841, 17.0576) (20.5924, 17.0475) knots -0.013599 -0.013599 -0.013599 -0.013599 -0.010706 -0.010706 -0.007813 -0.007813 -0.003906 -0.003906 0 0 0 0
  spline S165 degree 3 poles (21.6676, 19.018) (21.5153, 18.6782) (21.3439, 18.3387) (20.9889, 17.7295) (20.7975, 17.4368) (20.5907, 17.173) knots -0.220678 -0.220678 -0.220678 -0.220678 -0.107909 -0.107909 -0.008028 -0.008028 -0.008028 -0.008028
  arc A84 (21.6676, 19.018) -> (21.1787, 19.561) centre (0, 0) ccw
  spline S166 degree 3 poles (19.2312, 18.6828) (19.5152, 18.861) (19.8263, 19.0207) (20.4692, 19.31) (20.8249, 19.445) (21.1787, 19.561) knots -0.210627 -0.210627 -0.210627 -0.210627 -0.111696 -0.111696 0 0 0 0
  spline S167 degree 3 poles (19.1066, 18.6976) (19.1134, 18.6907) (19.1211, 18.6848) (19.1379, 18.6755) (19.147, 18.672) (19.1691, 18.6671) (19.1823, 18.6668) (19.2079, 18.6712) (19.2202, 18.6759) (19.2312, 18.6828) knots -0.013599 -0.013599 -0.013599 -0.013599 -0.010706 -0.010706 -0.007813 -0.007813 -0.003906 -0.003906 0 0 0 0
  arc A85 (19.1066, 18.6976) -> (18.6976, 19.1066) centre (0, 0) ccw
  spline S168 degree 3 poles (18.6828, 19.2312) (18.6777, 19.2231) (18.6738, 19.2142) (18.6686, 19.1956) (18.6674, 19.186) (18.6678, 19.1633) (18.6706, 19.1505) (18.6809, 19.1266) (18.6883, 19.1157) (18.6976, 19.1066) knots -0.013599 -0.013599 -0.013599 -0.013599 -0.010706 -0.010706 -0.007813 -0.007813 -0.003906 -0.003906 0 0 0 0
  spline S169 degree 3 poles (19.561, 21.1787) (19.445, 20.8249) (19.31, 20.4692) (19.0207, 19.8263) (18.861, 19.5152) (18.6828, 19.2312) knots -0.220678 -0.220678 -0.220678 -0.220678 -0.107909 -0.107909 -0.008028 -0.008028 -0.008028 -0.008028
  arc A86 (19.561, 21.1787) -> (19.018, 21.6676) centre (0, 0) ccw
  spline S170 degree 3 poles (17.173, 20.5907) (17.4368, 20.7975) (17.7295, 20.9889) (18.3387, 21.3439) (18.6782, 21.5153) (19.018, 21.6676) knots -0.210627 -0.210627 -0.210627 -0.210627 -0.111696 -0.111696 0 0 0 0
  spline S171 degree 3 poles (17.0475, 20.5924) (17.055, 20.5862) (17.0632, 20.5812) (17.081, 20.5736) (17.0904, 20.5711) (17.1129, 20.5686) (17.126, 20.5696) (17.151, 20.5767) (17.1628, 20.5827) (17.173, 20.5907) knots -0.013599 -0.013599 -0.013599 -0.013599 -0.010706 -0.010706 -0.007813 -0.007813 -0.003906 -0.003906 0 0 0 0
  arc A87 (17.0475, 20.5924) -> (16.598, 20.9564) centre (0, 0) ccw
  spline S172 degree 3 poles (16.5703, 21.0788) (16.566, 21.0701) (16.5631, 21.0609) (16.5599, 21.0419) (16.5597, 21.0322) (16.5624, 21.0097) (16.5665, 20.9972) (16.5793, 20.9745) (16.5878, 20.9645) (16.598, 20.9564) knots -0.013599 -0.013599 -0.013599 -0.013599 -0.010706 -0.010706 -0.007813 -0.007813 -0.003906 -0.003906 0 0 0 0
  spline S173 degree 3 poles (17.24, 23.1074) (17.1617, 22.7434) (17.0646, 22.3755) (16.8441, 21.7059) (16.7177, 21.3798) (16.5703, 21.0788) knots -0.220678 -0.220678 -0.220678 -0.220678 -0.107909 -0.107909 -0.008028 -0.008028 -0.008028 -0.008028
  arc A88 (17.24, 23.1074) -> (16.6489, 23.5368) centre (0, 0) ccw
  spline S174 degree 3 poles (14.9266, 22.273) (15.1674, 22.5063) (15.4385, 22.7272) (16.0071, 23.1439) (16.327, 23.3499) (16.6489, 23.5368) knots -0.210627 -0.210627 -0.210627 -0.210627 -0.111696 -0.111696 0 0 0 0
  spline S175 degree 3 poles (14.8017, 22.2615) (14.8097, 22.2562) (14.8184, 22.252) (14.8369, 22.2464) (14.8465, 22.2449) (14.8691, 22.2447) (14.882, 22.2471) (14.9062, 22.2568) (14.9173, 22.2639) (14.9266, 22.273) knots -0.013599 -0.013599 -0.013599 -0.013599 -0.010706 -0.010706 -0.007813 -0.007813 -0.003906 -0.003906 0 0 0 0
  arc A89 (14.8017, 22.2615) -> (14.3165, 22.5766) centre (0, 0) ccw
  spline S176 degree 3 poles (14.2762, 22.6954) (14.2729, 22.6863) (14.2709, 22.6768) (14.2697, 22.6576) (14.2705, 22.6479) (14.2756, 22.6258) (14.2809, 22.6138) (14.296, 22.5926) (14.3055, 22.5835) (14.3165, 22.5766) knots -0.013599 -0.013599 -0.013599 -0.013599 -0.010706 -0.010706 -0.007813 -0.007813 -0.003906 -0.003906 0 0 0 0
  spline S177 degree 3 poles (14.7302, 24.7828) (14.6904, 24.4127) (14.6323, 24.0367) (14.4829, 23.3477) (14.3914, 23.0102) (14.2762, 22.6954) knots -0.220678 -0.220678 -0.220678 -0.220678 -0.107909 -0.107909 -0.008028 -0.008028 -0.008028 -0.008028
  arc A90 (14.7302, 24.7828) -> (14.0975, 25.1482) centre (0, 0) ccw
  spline S178 degree 3 poles (12.5167, 23.7112) (12.7317, 23.9684) (12.9783, 24.2164) (13.5003, 24.6903) (13.7968, 24.9286) (14.0975, 25.1482) knots -0.210627 -0.210627 -0.210627 -0.210627 -0.111696 -0.111696 0 0 0 0
  spline S179 degree 3 poles (12.3936, 23.6868) (12.4022, 23.6823) (12.4113, 23.6791) (12.4302, 23.6754) (12.4399, 23.6749) (12.4625, 23.6771) (12.4751, 23.6808) (12.4981, 23.693) (12.5083, 23.7012) (12.5167, 23.7112) knots -0.013599 -0.013599 -0.013599 -0.013599 -0.010706 -0.010706 -0.007813 -0.007813 -0.003906 -0.003906 0 0 0 0
  arc A91 (12.3936, 23.6868) -> (11.8782, 23.9494) centre (0, 0) ccw
  spline S180 degree 3 poles (11.8257, 24.0633) (11.8233, 24.054) (11.8223, 24.0443) (11.8231, 24.025) (11.8249, 24.0155) (11.8323, 23.9941) (11.8389, 23.9827) (11.8561, 23.9632) (11.8665, 23.9552) (11.8782, 23.9494) knots -0.013599 -0.013599 -0.013599 -0.013599 -0.010706 -0.010706 -0.007813 -0.007813 -0.003906 -0.003906 0 0 0 0
  spline S181 degree 3 poles (12.059, 26.1868) (12.0581, 25.8145) (12.0396, 25.4345) (11.9631, 24.7337) (11.9073, 24.3884) (11.8257, 24.0633) knots -0.220678 -0.220678 -0.220678 -0.220678 -0.107909 -0.107909 -0.008028 -0.008028 -0.008028 -0.008028
  arc A92 (12.059, 26.1868) -> (11.3915, 26.484) centre (0, 0) ccw
  spline S182 degree 3 poles (9.9696, 24.8897) (10.1566, 25.1679) (10.3759, 25.4404) (10.8455, 25.9662) (11.1155, 26.2342) (11.3915, 26.484) knots -0.210627 -0.210627 -0.210627 -0.210627 -0.111696 -0.111696 0 0 0 0
  spline S183 degree 3 poles (9.8498, 24.8525) (9.8587, 24.8489) (9.8682, 24.8467) (9.8874, 24.845) (9.8971, 24.8455) (9.9193, 24.85) (9.9314, 24.8551) (9.9531, 24.8696) (9.9624, 24.8789) (9.9696, 24.8897) knots -0.013599 -0.013599 -0.013599 -0.013599 -0.010706 -0.010706 -0.007813 -0.007813 -0.003906 -0.003906 0 0 0 0
  arc A93 (9.8498, 24.8525) -> (9.3097, 25.0598) centre (0, 0) ccw
  spline S184 degree 3 poles (9.2456, 25.1676) (9.2442, 25.1581) (9.2442, 25.1484) (9.2471, 25.1293) (9.2499, 25.12) (9.2594, 25.0995) (9.2672, 25.0888) (9.2863, 25.0712) (9.2975, 25.0643) (9.3097, 25.0598) knots -0.013599 -0.013599 -0.013599 -0.013599 -0.010706 -0.010706 -0.007813 -0.007813 -0.003906 -0.003906 0 0 0 0
  spline S185 degree 3 poles (9.2557, 27.3039) (9.2937, 26.9335) (9.315, 26.5537) (9.3122, 25.8487) (9.2928, 25.4995) (9.2456, 25.1676) knots -0.220678 -0.220678 -0.220678 -0.220678 -0.107909 -0.107909 -0.008028 -0.008028 -0.008028 -0.008028
  arc A94 (9.2557, 27.3039) -> (8.5608, 27.5296) centre (0, 0) ccw
  spline S186 degree 3 poles (7.3133, 25.7954) (7.4702, 26.0917) (7.6598, 26.3856) (8.0719, 26.9576) (8.3124, 27.2523) (8.5608, 27.5296) knots -0.210627 -0.210627 -0.210627 -0.210627 -0.111696 -0.111696 0 0 0 0
  spline S187 degree 3 poles (7.198, 25.7459) (7.2073, 25.7433) (7.2169, 25.7421) (7.2362, 25.7424) (7.2458, 25.7439) (7.2674, 25.7508) (7.2789, 25.757) (7.2989, 25.7737) (7.3072, 25.7839) (7.3133, 25.7954) knots -0.013599 -0.013599 -0.013599 -0.013599 -0.010706 -0.010706 -0.007813 -0.007813 -0.003906 -0.003906 0 0 0 0
  arc A95 (7.198, 25.7459) -> (6.6393, 25.8956) centre (0, 0) ccw
  spline S188 degree 3 poles (6.5642, 25.9962) (6.5638, 25.9865) (6.5649, 25.9769) (6.5697, 25.9582) (6.5734, 25.9493) (6.5851, 25.9298) (6.5939, 25.9201) (6.6148, 25.9045) (6.6267, 25.8989) (6.6393, 25.8956) knots -0.013599 -0.013599 -0.013599 -0.013599 -0.010706 -0.010706 -0.007813 -0.007813 -0.003906 -0.003906 0 0 0 0
  spline S189 degree 3 poles (6.351, 28.1218) (6.4275, 27.7574) (6.4884, 27.3819) (6.5592, 26.6805) (6.5765, 26.3312) (6.5642, 25.9962) knots -0.220678 -0.220678 -0.220678 -0.220678 -0.107909 -0.107909 -0.008028 -0.008028 -0.008028 -0.008028
  arc A96 (6.351, 28.1218) -> (5.6363, 28.2737) centre (0, 0) ccw
  spline S190 degree 3 poles (4.5769, 26.4186) (4.702, 26.7296) (4.8598, 27.0417) (5.2098, 27.6537) (5.4182, 27.9719) (5.6363, 28.2737) knots -0.210627 -0.210627 -0.210627 -0.210627 -0.111696 -0.111696 0 0 0 0
  spline S191 degree 3 poles (4.4674, 26.3573) (4.4769, 26.3557) (4.4866, 26.3554) (4.5058, 26.3578) (4.5151, 26.3603) (4.5359, 26.3693) (4.5467, 26.3768) (4.5649, 26.3955) (4.572, 26.4065) (4.5769, 26.4186) knots -0.013599 -0.013599 -0.013599 -0.013599 -0.010706 -0.010706 -0.007813 -0.007813 -0.003906 -0.003906 0 0 0 0
  arc A97 (4.4674, 26.3573) -> (3.8961, 26.4478) centre (0, 0) ccw
  spline S192 degree 3 poles (3.8109, 26.5399) (3.8115, 26.5303) (3.8136, 26.5208) (3.8203, 26.5027) (3.825, 26.4942) (3.8386, 26.4761) (3.8484, 26.4674) (3.8708, 26.4541) (3.8832, 26.4497) (3.8961, 26.4478) knots -0.013599 -0.013599 -0.013599 -0.013599 -0.010706 -0.010706 -0.007813 -0.007813 -0.003906 -0.003906 0 0 0 0
  spline S193 degree 3 poles (3.3766, 28.6316) (3.4908, 28.2772) (3.5906, 27.9101) (3.7344, 27.2199) (3.7881, 26.8744) (3.8109, 26.5399) knots -0.220678 -0.220678 -0.220678 -0.220678 -0.107909 -0.107909 -0.008028 -0.008028 -0.008028 -0.008028
  arc A98 (3.3766, 28.6316) -> (2.65, 28.708) centre (0, 0) ccw
  spline S194 degree 3 poles (1.7903, 26.7523) (1.8822, 27.0747) (2.0065, 27.4015) (2.2907, 28.0467) (2.4646, 28.385) (2.65, 28.708) knots -0.210627 -0.210627 -0.210627 -0.210627 -0.111696 -0.111696 0 0 0 0
  spline S195 degree 3 poles (1.6879, 26.6799) (1.6975, 26.6793) (1.7071, 26.68) (1.7259, 26.6844) (1.735, 26.6879) (1.7547, 26.699) (1.7647, 26.7076) (1.7808, 26.728) (1.7868, 26.7397) (1.7903, 26.7523) knots -0.013599 -0.013599 -0.013599 -0.013599 -0.010706 -0.010706 -0.007813 -0.007813 -0.003906 -0.003906 0 0 0 0
  arc A99 (1.6879, 26.6799) -> (1.1102, 26.7101) centre (0, 0) ccw
  spline S196 degree 3 poles (1.0158, 26.7929) (1.0175, 26.7834) (1.0205, 26.7741) (1.0291, 26.7569) (1.0346, 26.7489) (1.0501, 26.7323) (1.0607, 26.7246) (1.0844, 26.7138) (1.0972, 26.7107) (1.1102, 26.7101) knots -0.013599 -0.013599 -0.013599 -0.013599 -0.010706 -0.010706 -0.007813 -0.007813 -0.003906 -0.003906 0 0 0 0
  spline S197 degree 3 poles (0.3653, 28.8277) (0.5159, 28.4872) (0.6536, 28.1325) (0.8687, 27.4612) (0.9582, 27.1231) (1.0158, 26.7929) knots -0.220678 -0.220678 -0.220678 -0.220678 -0.107909 -0.107909 -0.008028 -0.008028 -0.008028 -0.008028
  arc A100 (0.3653, 28.8277) -> (-0.3653, 28.8277) centre (0, 0) ccw
  spline S198 degree 3 poles (-1.0158, 26.7929) (-0.9582, 27.1231) (-0.8687, 27.4612) (-0.6536, 28.1325) (-0.5159, 28.4872) (-0.3653, 28.8277) knots -0.210627 -0.210627 -0.210627 -0.210627 -0.111696 -0.111696 0 0 0 0
  spline S199 degree 3 poles (-1.1102, 26.7101) (-1.1006, 26.7105) (-1.091, 26.7123) (-1.0728, 26.7186) (-1.0642, 26.723) (-1.0457, 26.7362) (-1.0367, 26.7457) (-1.0228, 26.7678) (-1.0181, 26.78) (-1.0158, 26.7929) knots -0.013599 -0.013599 -0.013599 -0.013599 -0.010706 -0.010706 -0.007813 -0.007813 -0.003906 -0.003906 0 0 0 0
  arc A101 (-1.1102, 26.7101) -> (-1.6879, 26.6799) centre (0, 0) ccw
  spline S200 degree 3 poles (-1.7903, 26.7523) (-1.7877, 26.743) (-1.7837, 26.7341) (-1.7734, 26.7179) (-1.7671, 26.7105) (-1.75, 26.6957) (-1.7386, 26.6891) (-1.7139, 26.6808) (-1.7008, 26.679) (-1.6879, 26.6799) knots -0.013599 -0.013599 -0.013599 -0.013599 -0.010706 -0.010706 -0.007813 -0.007813 -0.003906 -0.003906 0 0 0 0
  spline S201 degree 3 poles (-2.65, 28.708) (-2.4646, 28.385) (-2.2907, 28.0467) (-2.0065, 27.4015) (-1.8822, 27.0747) (-1.7903, 26.7523) knots -0.220678 -0.220678 -0.220678 -0.220678 -0.107909 -0.107909 -0.008028 -0.008028 -0.008028 -0.008028
  arc A102 (-2.65, 28.708) -> (-3.3766, 28.6316) centre (0, 0) ccw
  spline S202 degree 3 poles (-3.8109, 26.5399) (-3.7881, 26.8744) (-3.7344, 27.2199) (-3.5906, 27.9101) (-3.4908, 28.2772) (-3.3766, 28.6316) knots -0.210627 -0.210627 -0.210627 -0.210627 -0.111696 -0.111696 0 0 0 0
  spline S203 degree 3 poles (-3.8961, 26.4478) (-3.8865, 26.4492) (-3.8773, 26.452) (-3.8598, 26.4601) (-3.8517, 26.4654) (-3.8347, 26.4804) (-3.8267, 26.4908) (-3.8152, 26.5142) (-3.8118, 26.5269) (-3.8109, 26.5399) knots -0.013599 -0.013599 -0.013599 -0.013599 -0.010706 -0.010706 -0.007813 -0.007813 -0.003906 -0.003906 0 0 0 0
  arc A103 (-3.8961, 26.4478) -> (-4.4674, 26.3573) centre (0, 0) ccw
  spline S204 degree 3 poles (-4.5769, 26.4186) (-4.5733, 26.4096) (-4.5684, 26.4012) (-4.5564, 26.3861) (-4.5494, 26.3795) (-4.5308, 26.3665) (-4.5188, 26.3612) (-4.4934, 26.3555) (-4.4803, 26.3551) (-4.4674, 26.3573) knots -0.013599 -0.013599 -0.013599 -0.013599 -0.010706 -0.010706 -0.007813 -0.007813 -0.003906 -0.003906 0 0 0 0
  spline S205 degree 3 poles (-5.6363, 28.2737) (-5.4182, 27.9719) (-5.2098, 27.6537) (-4.8598, 27.0417) (-4.702, 26.7296) (-4.5769, 26.4186) knots -0.220678 -0.220678 -0.220678 -0.220678 -0.107909 -0.107909 -0.008028 -0.008028 -0.008028 -0.008028
  arc A104 (-5.6363, 28.2737) -> (-6.351, 28.1218) centre (0, 0) ccw
  spline S206 degree 3 poles (-6.5642, 25.9962) (-6.5765, 26.3312) (-6.5592, 26.6805) (-6.4884, 27.3819) (-6.4275, 27.7574) (-6.351, 28.1218) knots -0.210627 -0.210627 -0.210627 -0.210627 -0.111696 -0.111696 0 0 0 0
  spline S207 degree 3 poles (-6.6393, 25.8956) (-6.6299, 25.898) (-6.621, 25.9018) (-6.6045, 25.9117) (-6.5969, 25.9178) (-6.5816, 25.9345) (-6.5748, 25.9457) (-6.5658, 25.9702) (-6.5637, 25.9831) (-6.5642, 25.9962) knots -0.013599 -0.013599 -0.013599 -0.013599 -0.010706 -0.010706 -0.007813 -0.007813 -0.003906 -0.003906 0 0 0 0
  arc A105 (-6.6393, 25.8956) -> (-7.198, 25.7459) centre (0, 0) ccw
  spline S208 degree 3 poles (-7.3133, 25.7954) (-7.3088, 25.7869) (-7.3031, 25.7791) (-7.2896, 25.7653) (-7.2819, 25.7594) (-7.2621, 25.7485) (-7.2495, 25.7444) (-7.2237, 25.7414) (-7.2106, 25.7424) (-7.198, 25.7459) knots -0.013599 -0.013599 -0.013599 -0.013599 -0.010706 -0.010706 -0.007813 -0.007813 -0.003906 -0.003906 0 0 0 0
  spline S209 degree 3 poles (-8.5608, 27.5296) (-8.3124, 27.2523) (-8.0719, 26.9576) (-7.6598, 26.3856) (-7.4702, 26.0917) (-7.3133, 25.7954) knots -0.220678 -0.220678 -0.220678 -0.220678 -0.107909 -0.107909 -0.008028 -0.008028 -0.008028 -0.008028
  arc A106 (-8.5608, 27.5296) -> (-9.2557, 27.3039) centre (0, 0) ccw
  spline S210 degree 3 poles (-9.2456, 25.1676) (-9.2928, 25.4995) (-9.3122, 25.8487) (-9.315, 26.5537) (-9.2937, 26.9335) (-9.2557, 27.3039) knots -0.210627 -0.210627 -0.210627 -0.210627 -0.111696 -0.111696 0 0 0 0
  spline S211 degree 3 poles (-9.3097, 25.0598) (-9.3007, 25.0631) (-9.2922, 25.0678) (-9.2768, 25.0794) (-9.27, 25.0863) (-9.2565, 25.1045) (-9.2508, 25.1163) (-9.2444, 25.1416) (-9.2437, 25.1547) (-9.2456, 25.1676) knots -0.013599 -0.013599 -0.013599 -0.013599 -0.010706 -0.010706 -0.007813 -0.007813 -0.003906 -0.003906 0 0 0 0
  arc A107 (-9.3097, 25.0598) -> (-9.8498, 24.8525) centre (0, 0) ccw
  spline S212 degree 3 poles (-9.9696, 24.8897) (-9.9642, 24.8817) (-9.9577, 24.8745) (-9.9429, 24.8622) (-9.9346, 24.8572) (-9.9137, 24.8483) (-9.9008, 24.8456) (-9.8748, 24.8453) (-9.8619, 24.8477) (-9.8498, 24.8525) knots -0.013599 -0.013599 -0.013599 -0.013599 -0.010706 -0.010706 -0.007813 -0.007813 -0.003906 -0.003906 0 0 0 0
  spline S213 degree 3 poles (-11.3915, 26.484) (-11.1155, 26.2342) (-10.8455, 25.9662) (-10.3759, 25.4404) (-10.1566, 25.1679) (-9.9696, 24.8897) knots -0.220678 -0.220678 -0.220678 -0.220678 -0.107909 -0.107909 -0.008028 -0.008028 -0.008028 -0.008028
  arc A108 (-11.3915, 26.484) -> (-12.059, 26.1868) centre (0, 0) ccw
  spline S214 degree 3 poles (-11.8257, 24.0633) (-11.9073, 24.3884) (-11.9631, 24.7337) (-12.0396, 25.4345) (-12.0581, 25.8145) (-12.059, 26.1868) knots -0.210627 -0.210627 -0.210627 -0.210627 -0.111696 -0.111696 0 0 0 0
  spline S215 degree 3 poles (-11.8782, 23.9494) (-11.8696, 23.9537) (-11.8616, 23.9592) (-11.8475, 23.9723) (-11.8414, 23.9799) (-11.8299, 23.9994) (-11.8255, 24.0118) (-11.8218, 24.0376) (-11.8225, 24.0507) (-11.8257, 24.0633) knots -0.013599 -0.013599 -0.013599 -0.013599 -0.010706 -0.010706 -0.007813 -0.007813 -0.003906 -0.003906 0 0 0 0
  arc A109 (-11.8782, 23.9494) -> (-12.1366, 23.8195) centre (0, 0) ccw
  circle A110 centre (0, 0) radius 8
  circle A111 centre (0, 0) radius 10
  circle A112 centre (0, 0) radius 25
  line L2 (0, -40) -> (0, 0)
  line L3 (34.641, -20) -> (0, 0)
  line L4 (34.641, 20) -> (0, 0)
  line L5 (0, 40) -> (0, 0)
  line L6 (-34.641, 20) -> (0, 0)
  line L7 (-34.641, -20) -> (0, 0)
  dimension "d73" = 20
  dimension "d75" = 360
  constraint coincident A0.centre A1.centre
  constraint vertical L2
  measures "d73" diameter of A111
extrude "Estrusione9" cut sketch "Schizzo7" against normal blind 1 contours A0 A111 A112 L5 L6 | A111 A112 L3 L4 | A111 A112 L2 L7 in component "Spur Gear (60 teeth) (1)"
sketch "Schizzo9" plane through (0, 0, 2) normal (0, 0, 1) x (-1, 0, 0)
  line L0 (8.6603, -5) -> (21.6506, -12.5)
  arc A0 (21.6506, -12.5) -> (21.6506, 12.5) centre (0, 0) ccw
  line L1 (21.6506, 12.5) -> (8.6603, 5)
  arc A1 (8.6603, -5) -> (8.6603, 5) centre (0, 0) ccw
  line L2 (7.9146, 3.8207) -> (7.9146, -14.1793) construction
  line L3 (7.9146, -14.1793) -> (20.9146, -14.1793) construction
  line L4 (20.9146, -14.1793) -> (20.9146, 3.8207) construction
  line L5 (20.9146, 3.8207) -> (7.9146, 3.8207) construction
  dimension "d78" = 5
  text T0 "2h" font "Arial" height 5 bold align left top in box 18 x 13 at (7.9146, 3.8207) x (0, -1) y (1, 0) spacing 1 kerned